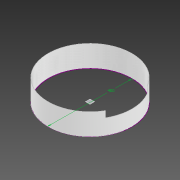
# Autodesk Inventor part: border
Saved by Autodesk Inventor 2020 (Build 240168000, 168)
## iProperties
Created: 2022-08-25
Part Number: border
Material: PC/ABS Plastic
Document SubType Name: Modeling
Designer: Umair
Density: 0.357273 g/cm^3
Appearance: Smooth - White
Author: Umair
Autodesk Inventor part; units mm, degrees
ref_plane "YZ Plane" through (0, 0, 0) normal (1, 0, 0) x (0, 1, 0)
ref_plane "XZ Plane" through (0, 0, 0) normal (0, 1, 0) x (-1, 0, 0)
ref_plane "XY Plane" through (0, 0, 0) normal (0, 0, 1) x (1, 0, 0)
sketch "Sketch1" plane through (0, 0, 0) normal (0, 1, 0) x (-1, 0, 0)
  circle A0 centre (0, 0) radius 200
  dimension "d0" = 400
  constraints: 1 centre point, 1 coincident
  measures "d0" diameter of A0
ref_plane "Work Plane1" through (0, 3, 0) normal (0, 1, 0) x (1, 0, 0)
sketch "Sketch2" plane through (0, 3, 0) normal (0, 1, 0) x (1, 0, 0)
  line L0 (-63.5, -143.5) -> (63.5, -143.5)
  line L1 (63.5, -143.5) -> (63.5, 143.5)
  line L2 (63.5, 143.5) -> (-63.5, 143.5)
  line L3 (-63.5, 143.5) -> (-63.5, -143.5)
  line L4 (-63.5, -143.5) -> (63.5, 143.5) construction
  line L5 (63.5, -143.5) -> (-63.5, 143.5) construction
  point P0 (0, 0)
  dimension "d3" = 127
  dimension "d4" = 287
  constraints: 12 end point, 2 midpoint, 2 parallel, 1 horizontal, 1 perpendicular
  measures "d3" distance of L2.end L1.end
  measures "d4" distance of L1.end L0.end
extrude "Extrusion2" [suppressed]
ref_plane "Work Plane4" through (0, 3, 0) normal (0, 1, 0) x (1, 0, 0)
sketch "Sketch3" plane through (0, 3, 0) normal (0, 1, 0) x (1, 0, 0)
  line L0 (-63.5, 143.5) -> (-63.5, -143.5) projected
  line L1 (-63.5, 0) -> (-123.5, 0)
  line L2 (-123.5, 0) -> (-93.5, 0)
  line L3 (-93.5, 0) -> (-119.5, 0)
  circle A0 centre (-119.5, 0) radius 2.5
  circle A1 centre (-117.932, -8.8925) radius 2.5
  circle A2 centre (-113.4172, -16.7125) radius 2.5
  circle A3 centre (-106.5, -22.5167) radius 2.5
  circle A4 centre (-98.0149, -25.605) radius 2.5
  circle A5 centre (-88.9851, -25.605) radius 2.5
  circle A6 centre (-80.5, -22.5167) radius 2.5
  circle A7 centre (-73.5828, -16.7125) radius 2.5
  circle A8 centre (-69.068, -8.8925) radius 2.5
  circle A9 centre (-67.5, 0) radius 2.5
  circle A10 centre (-69.068, 8.8925) radius 2.5
  circle A11 centre (-73.5828, 16.7125) radius 2.5
  circle A12 centre (-80.5, 22.5167) radius 2.5
  circle A13 centre (-88.9851, 25.605) radius 2.5
  circle A14 centre (-98.0149, 25.605) radius 2.5
  circle A15 centre (-106.5, 22.5167) radius 2.5
  circle A16 centre (-113.4172, 16.7125) radius 2.5
  circle A17 centre (-117.932, 8.8925) radius 2.5
  line L4 (-93.5, 0) -> (-110.5, 0)
  line L5 (-110.5, 0) -> (-92.5712, 0)
  line L6 (-93.5, 0) -> (-103.5, 0)
  circle A18 centre (-110.5, 0) radius 2
  circle A19 centre (-103.5, 0) radius 1.5
  circle A20 centre (-109.4748, -5.8143) radius 2
  circle A21 centre (-106.5228, -10.9274) radius 2
  circle A22 centre (-102, -14.7224) radius 2
  circle A23 centre (-96.452, -16.7417) radius 2
  circle A24 centre (-90.548, -16.7417) radius 2
  circle A25 centre (-85, -14.7224) radius 2
  circle A26 centre (-80.4772, -10.9274) radius 2
  circle A27 centre (-77.5252, -5.8143) radius 2
  circle A28 centre (-76.5, 0) radius 2
  circle A29 centre (-77.5252, 5.8143) radius 2
  circle A30 centre (-80.4772, 10.9274) radius 2
  circle A31 centre (-85, 14.7224) radius 2
  circle A32 centre (-90.548, 16.7417) radius 2
  circle A33 centre (-96.452, 16.7417) radius 2
  circle A34 centre (-102, 14.7224) radius 2
  circle A35 centre (-106.5228, 10.9274) radius 2
  circle A36 centre (-109.4748, 5.8143) radius 2
  circle A37 centre (-101.5902, -5.8779) radius 1.5
  circle A38 centre (-96.5902, -9.5106) radius 1.5
  circle A39 centre (-90.4098, -9.5106) radius 1.5
  circle A40 centre (-85.4098, -5.8779) radius 1.5
  circle A41 centre (-83.5, 0) radius 1.5
  circle A42 centre (-85.4098, 5.8779) radius 1.5
  circle A43 centre (-90.4098, 9.5106) radius 1.5
  circle A44 centre (-96.5902, 9.5106) radius 1.5
  circle A45 centre (-101.5902, 5.8779) radius 1.5
  point P0 (0, 0)
  dimension "d7" = 60
  dimension "d8" = 30
  dimension "d9" = 26
  dimension "d10" = 5
  dimension "d13" = 360
  dimension "d15" = 17
  dimension "d16" = 10
  dimension "d18" = 4
  dimension "d19" = 3
  dimension "d22" = 360
  dimension "d26" = 360
  constraints: 46 centre point, 12 end point, 4 point on line, 3 coincident, 2 midpoint, 1 horizontal, 95 other
  measures "d7" distance of L1.start L1.end
  measures "d8" distance of L1.end L2.end
  measures "d9" distance of L2.end L3.end
  measures "d10" diameter of A0
  measures "d15" distance of L2.end L4.end
  measures "d16" distance of L2.end L6.end
  measures "d18" diameter of A18
  measures "d19" diameter of A19
extrude "Extrusion3" [suppressed]
ref_plane "Work Plane2" through (0, 3, 0) normal (0, 1, 0) x (1, 0, 0)
sketch "Sketch4" plane through (0, 3, 0) normal (0, 1, 0) x (1, 0, 0)
  line L0 (0, 0) -> (0, -170)
  line L1 (0, -170) -> (0, 170)
  line L2 (0, -170) -> (-40, -170)
  line L3 (-40, -170) -> (-65, -170)
  line L4 (-65, -170) -> (0, -170)
  line L5 (0, -170) -> (65, -170)
  line L6 (0, 170) -> (-65, 170)
  line L7 (-65, 170) -> (0, 170)
  line L8 (0, 170) -> (65, 170)
  circle A0 centre (65, 170) radius 1.5
  circle A1 centre (-65, 170) radius 1.5
  circle A2 centre (-65, -170) radius 1.5
  circle A3 centre (65, -170) radius 1.5
  dimension "d30" = 170
  dimension "d31" = 340
  dimension "d32" = 40
  dimension "d33" = 25
  dimension "d34" = 65
  dimension "d35" = 65
  dimension "d36" = 65
  dimension "d37" = 65
  dimension "d38" = 65
  dimension "d39" = 3
  dimension "d40" = 3
  dimension "d41" = 3
  dimension "d42" = 3
  constraints: 18 end point, 4 centre point, 4 coincident, 4 point on line, 2 collinear, 2 horizontal, 1 vertical
  measures "d30" distance of L0.start L0.end
  measures "d31" distance of L0.end L1.end
  measures "d32" distance of L0.end L2.end
  measures "d33" distance of L2.end L3.end
  measures "d34" distance of L3.end L0.end
  measures "d35" distance of L0.end L5.end
  measures "d36" distance of L1.end L6.end
  measures "d37" distance of L6.end L1.end
  measures "d38" distance of L1.end L8.end
  measures "d39" diameter of A0
  measures "d40" diameter of A1
  measures "d41" diameter of A2
  measures "d42" diameter of A3
extrude "Extrusion4" [suppressed]
ref_plane "Work Plane3" through (0, 3, 0) normal (0, 1, 0) x (1, 0, 0)
sketch "Sketch5" plane through (0, 3, 0) normal (0, 1, 0) x (1, 0, 0)
  circle A0 centre (0, 0) radius 201
  circle A1 centre (0, 0) radius 200
  dimension "d45" = 402
  dimension "d46" = 400
  constraints: 2 centre point, 2 coincident
  measures "d45" diameter of A0
  measures "d46" diameter of A1
extrude "Extrusion5" add sketch "Sketch5" along normal blind 100 and the other way blind 3
sketch "Sketch6" plane through (0, 0, 0) normal (1, 0, 0) x (0, 1, 0)
  line L0 (0, -200) -> (0, 200) projected
  line L1 (0, -200) -> (0, 200)
  line L2 (0, 200) -> (103, 201)
  line L3 (0, 201) -> (103, 201) projected
  line L4 (103, -201) -> (103, 201) projected
  line L5 (103, -201) -> (103, 201)
  line L6 (103, 201) -> (103, 0)
  line L7 (73, -100) -> (133, -100)
  line L8 (133, -100) -> (133, 100)
  line L9 (133, 100) -> (73, 100)
  line L10 (73, 100) -> (73, -100)
  line L11 (73, -100) -> (133, 100) construction
  line L12 (133, -100) -> (73, 100) construction
  point P0 (0, 0)
  dimension "d51" = 60
  dimension "d52" = 200
  constraints: 20 end point, 4 equal length, 3 midpoint, 1 horizontal, 1 perpendicular, 1 point on line
  measures "d51" distance of L9.end L8.end
  measures "d52" distance of L8.end L7.end
extrude "Extrusion6" cut sketch "Sketch6" along normal blind 300
body "Solid1"
